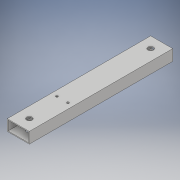
# Autodesk Inventor part: arm
Saved by Autodesk Inventor 2018 (Build 220112000, 112)
## iProperties
Created: 2020-01-22
Part Number: arm
Material: Generic
Document SubType Name: Modeling
Designer: s-2513225
Density: 1 g/cm^3
Appearance: Default
Author: s-2513225
Autodesk Inventor part; units mm, degrees
ref_plane "YZ Plane" through (0, 0, 0) normal (1, 0, 0) x (0, 1, 0)
ref_plane "XZ Plane" through (0, 0, 0) normal (0, 1, 0) x (-1, 0, 0)
ref_plane "XY Plane" through (0, 0, 0) normal (0, 0, 1) x (1, 0, 0)
sketch "Sketch1" plane through (0, 0, 0) normal (0, 0, 1) x (1, 0, 0)
  line L0 (0, 0) -> (50.8, 0)
  line L1 (50.8, 0) -> (50.8, 25.4)
  line L2 (50.8, 25.4) -> (0, 25.4)
  line L3 (0, 25.4) -> (0, 0)
  line L4 (1.905, 23.495) -> (48.895, 23.495)
  line L5 (48.895, 23.495) -> (48.895, 1.905)
  line L6 (48.895, 1.905) -> (1.905, 1.905)
  line L7 (1.905, 1.905) -> (1.905, 23.495)
  dimension "d0" = 50.8
  dimension "d1" = 25.4
  dimension "d2" = 1.905
  constraints: 16 end point, 4 parallel, 2 perpendicular, 1 horizontal, 3 other
  measures "d0" distance of L2.end L1.end
  measures "d1" distance of L1.end L0.end
  measures "d2" distance between parallel lines of L2 L4
extrude "Extrusion1" add sketch "Sketch1" along normal blind 330.2
sketch "Sketch2" plane through (0, 25.4, 0) normal (0, 1, 0) x (1, 0, 0)
  line L0 (1.905, -330.2) -> (48.895, -330.2) construction
  line L1 (25.4, -330.2) -> (25.4, -304.8) construction
  line L2 (25.4, -304.8) -> (25.4, -228.6) construction
  line L3 (50.8, 0) -> (0, 0) construction
  line L4 (25.4, 0) -> (25.4, -25.4) construction
  circle A0 centre (25.4, -304.8) radius 6.35
  circle A1 centre (25.4, -25.4) radius 6.35
  line L5 (25.4, -228.6) -> (12.7, -228.6) construction
  line L6 (12.7, -228.6) -> (25.4, -228.6) construction
  line L7 (25.4, -228.6) -> (38.1, -228.6) construction
  circle A2 centre (12.7, -228.6) radius 2.5797
  circle A3 centre (38.1, -228.6) radius 2.5797
  dimension "d5" = 25.4
  dimension "d6" = 76.2
  dimension "d7" = 25.4
  dimension "d8" = 12.7
  dimension "d9" = 12.7
  dimension "d10" = 12.7
  dimension "d11" = 12.7
  dimension "d12" = 5.1594
  dimension "d13" = 5.1594
  constraints: 12 end point, 4 centre point, 4 coincident, 2 midpoint, 2 point on line, 2 vertical, 1 collinear, 1 horizontal
  measures "d5" distance of L1.start L1.end
  measures "d6" distance of L1.end L2.end
  measures "d7" distance of L4.start L4.end
  measures "d8" diameter of A0
  measures "d9" diameter of A1
  measures "d10" distance of L2.end L5.end
  measures "d11" distance of L2.end L7.end
  measures "d12" diameter of A2
  measures "d13" diameter of A3
extrude "Extrusion2" cut sketch "Sketch2" against normal blind 355.6
body "Solid1"
